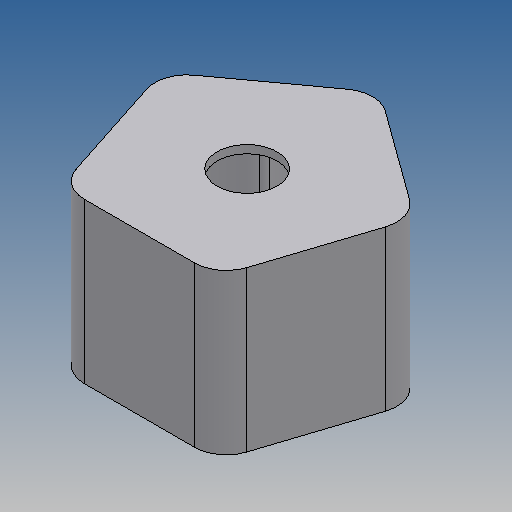
# Autodesk Inventor part: 21700_case
Saved by Autodesk Inventor 2019.4 (Build 234330000, 330)
## iProperties
Part Number: 21700_case
Material: GEDA Stahl
Document SubType Name: Modeling
Designer: Admin
Mass: 194.805 g
Surface Area: 199.588 cm^2
Volume: 24.7843 cm^3
Density: 7.86 g/cm^3
Appearance: GEDA Stahl A
Gewicht: 0,195 kg
G_L: 0
G_H: 0
G_B: 0
InventorVersion: 2019.4
VAULT_Status: in Bearbeitung
Revision: -
Max. Breite: 0
Max. Höhe: 0
Max. Länge: 0
Max. Abmessungen: 0 x 0 x 0
Volumen: 24784,336
Author: Admin
Autodesk Inventor part; units mm, degrees
note: some values were not read from the file. Left out: dimensions or parameters whose unit could not be read.
ref_plane "YZ Plane" through (0, 0, 0) normal (1, 0, 0) x (0, 1, 0)
ref_plane "XZ Plane" through (0, 0, 0) normal (0, 1, 0) x (-1, 0, 0)
ref_plane "XY Plane" through (0, 0, 0) normal (0, 0, 1) x (1, 0, 0)
sketch "Skizze1" plane through (0, 0, 0) normal (0, 0, 1) x (1, 0, 0)
  circle A0 centre (0, 0) radius 17.8637 construction
  circle A1 centre (-16.9894, 5.5202) radius 10.5 construction
  circle A2 centre (0, 17.8637) radius 10.5 construction
  circle A3 centre (16.9894, 5.5202) radius 10.5 construction
  circle A4 centre (10.5, -14.452) radius 10.5 construction
  circle A5 centre (-10.5, -14.452) radius 10.5 construction
  arc A6 (-10.4219, 14.3445) -> (-16.8629, -5.4791) centre (-16.9894, 5.5202) ccw
  arc A7 (10.4219, 14.3445) -> (-10.4219, 14.3445) centre (0, 17.8637) ccw
  arc A8 (16.8629, -5.4791) -> (10.4219, 14.3445) centre (16.9894, 5.5202) ccw
  arc A9 (0, -17.7307) -> (16.8629, -5.4791) centre (10.5, -14.452) ccw
  arc A10 (-16.8629, -5.4791) -> (0, -17.7307) centre (-10.5, -14.452) ccw
  line L0 (0, 33.3145) -> (31.684, 10.2948)
  line L1 (31.684, 10.2948) -> (19.5818, -26.952)
  line L2 (19.5818, -26.952) -> (-19.5818, -26.952)
  line L3 (-19.5818, -26.952) -> (-31.684, 10.2948)
  line L4 (-31.684, 10.2948) -> (0, 33.3145)
  dimension "d0" = 21
  dimension "d1" = 11
  dimension "d2" = 12.5
  constraints: 15 point on circle, 13 equal radius, 11 centre point, 10 end point, 7 coincident, 2 vertical alignment, 11 other
  measures "d0" diameter of A1
  measures "d1" radius of A7
  measures "d2" distance from line of A7.centre L4
extrude "Extrusion1" add sketch "Skizze1" along normal blind 38
fillet "Rundung1" radius 1 5 edges at (-10.4219, 14.3445, 19) (10.4219, 14.3445, 19) (16.8629, -5.4791, 19) (0, -17.7307, 19) (-16.8629, -5.4791, 19)
fillet "Rundung1" radius 8 5 edges at (19.5818, -26.952, 19) (31.684, 10.2948, 19) (0, 33.3145, 19) (-31.684, 10.2948, 19) (-19.5818, -26.952, 19)
sketch "Skizze2" plane through (0, 0, 38) normal (0, 0, 1) x (1, 0, 0)
  arc A0 (-21.3779, -21.4241) -> (-13.7694, -26.952) centre (-13.7694, -18.952) ccw projected
  line L0 (-13.7694, -26.952) -> (13.7694, -26.952) projected
  arc A1 (13.7694, -26.952) -> (21.3779, -21.4241) centre (13.7694, -18.952) ccw projected
  line L1 (21.3779, -21.4241) -> (29.8879, 4.7669) projected
  arc A2 (29.8879, 4.7669) -> (26.9817, 13.7112) centre (22.2794, 7.239) ccw projected
  line L2 (26.9817, 13.7112) -> (4.7023, 29.8981) projected
  arc A3 (4.7023, 29.8981) -> (-4.7023, 29.8981) centre (0, 23.426) ccw projected
  line L3 (-4.7023, 29.8981) -> (-26.9817, 13.7112) projected
  arc A4 (-26.9817, 13.7112) -> (-29.8879, 4.7669) centre (-22.2794, 7.239) ccw projected
  line L4 (-29.8879, 4.7669) -> (-21.3779, -21.4241) projected
  arc A5 (-18.539, -6.9437) -> (-19.0798, -5.2794) centre (-19.2698, -6.2611) ccw projected
  arc A6 (-12.3327, 15.4859) -> (-19.0798, -5.2794) centre (-16.9894, 5.5202) ccw projected
  arc A7 (-12.3327, 15.4859) -> (-10.917, 16.5145) centre (-11.9094, 16.3919) ccw projected
  arc A8 (10.917, 16.5145) -> (-10.917, 16.5145) centre (0, 17.8637) ccw projected
  arc A9 (10.917, 16.5145) -> (12.3327, 15.4859) centre (11.9094, 16.3919) ccw projected
  arc A10 (19.0798, -5.2794) -> (12.3327, 15.4859) centre (16.9894, 5.5202) ccw projected
  arc A11 (19.0798, -5.2794) -> (18.539, -6.9437) centre (19.2698, -6.2611) ccw projected
  arc A12 (0.875, -19.7774) -> (18.539, -6.9437) centre (10.5, -14.452) ccw projected
  arc A13 (0.875, -19.7774) -> (-0.875, -19.7774) centre (0, -20.2615) ccw projected
  arc A14 (-18.539, -6.9437) -> (-0.875, -19.7774) centre (-10.5, -14.452) ccw projected
  circle A15 centre (0, 0) radius 7.5
  dimension "d7" = 15
  constraints: 1 centre point, 1 coincident
  measures "d7" diameter of A15
extrude "Extrusion2" add sketch "Skizze2" along normal blind 2 contours L4 A4 L3 A3 L2 A2 L1 A1 L0 A0 | A5 A6 A7 A8 A9 A10 A11 A12 A13 A14
equation "\"G_L\" = 0"
equation "\"G_H\" = 0"
equation "\"G_B\" = 0"
